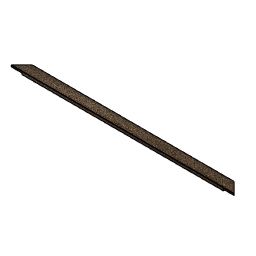
Top_Long (Autodesk Fusion 360 design; units mm, degrees)
Autodesk Fusion 360 part; units mm, degrees
sketch "Sketch1" plane through (0, 0, 0) normal (0, 0, 1) x (1, 0, 0)
  line L0 (914.4, 44.45) -> (914.4, -44.45) construction
  line L1 (914.4, -44.45) -> (-914.4, -44.45)
  line L2 (-914.4, -44.45) -> (-914.4, 44.45) construction
  line L3 (-914.4, 44.45) -> (914.4, -44.45) construction
  line L4 (914.4, 44.45) -> (-914.4, -44.45) construction
  line L5 (-914.4, -44.45) -> (-825.5, 44.45)
  line L6 (914.4, -44.45) -> (825.5, 44.45)
  line L7 (-914.4, 44.45) -> (-825.5, 44.45) construction
  line L8 (825.5, 44.45) -> (914.4, 44.45) construction
  line L9 (-825.5, 44.45) -> (825.5, 44.45)
  line L10 (0, 0) -> (0, -44.45) construction
  dimension "d27" = 1828.8
  dimension "d40" = 45
  dimension "d41" = 45
  dimension "d42" = 88.9
  constraint horizontal L7
  constraint perpendicular L0 L7
  constraint parallel L1 L7
  constraint parallel L0 L2
  constraint coincident L3 L10.start
  constraint coincident L4 L10.start
  constraint coincident L10.start origin
  constraint coincident L6.end L7
  constraint midpoint L1 L10.end
  constraint perpendicular L1 L10
  measures "d27" distance of L0.end L1.end
  measures "d40" angle of L1 L5
  measures "d41" angle of L1 L6
  measures "d42" distance of L1 L9
extrude "Extrude1" add sketch "Sketch1" along normal blind 25.4
sketch "Sketch9" plane through (0, 0, 0) normal (0, 0, 1) x (-1, 0, 0)
  line L0 (825.5, -44.45) -> (914.4, 44.45)
  line L1 (914.4, 44.45) -> (-914.4, 44.45)
  line L2 (-914.4, 44.45) -> (-825.5, -44.45)
  line L3 (914.4, 44.45) -> (825.5, -44.45)
  line L4 (825.5, -44.45) -> (825.5, 44.45)
  line L5 (825.5, 44.45) -> (914.4, 44.45)
  line L6 (-825.5, -44.45) -> (-914.4, 44.45)
  line L7 (-825.5, -44.45) -> (-825.5, 44.45)
  line L8 (-825.5, 44.45) -> (-914.4, 44.45)
  line L9 (-825.5, -44.45) -> (825.5, -44.45)
  line L10 (-825.5, -44.45) -> (-914.4, 44.45)
  line L11 (-914.4, 44.45) -> (914.4, 44.45)
  line L12 (914.4, 44.45) -> (825.5, -44.45)
  line L13 (825.5, -44.45) -> (-825.5, -44.45)
  constraint coincident L0.end L1.start
  constraint coincident L0.start L3.end
  constraint coincident L1 L4.end
  constraint perpendicular L1 L4
  constraint coincident L2.end L6.start
  constraint coincident L1.end L2.start
  constraint coincident L1 L7.end
  constraint perpendicular L1 L7
extrude "Extrude8" cut sketch "Sketch9" along normal blind 12.7 contours L0 L1 L3 L4 L5 L11 L12 | L1 L2 L6 L7 L8 L10 L11
chamfer "Chamfer2" distance 1.5875 angle 45 5 edges at (0, -44.45, 25.4) (0, -44.45, 0) (0, 44.45, 25.4) (914.4, -44.45, 19.05) (-914.4, -44.45, 19.05)
sketch "Sketch11" plane through (0, 44.45, 0) normal (0, 1, 0) x (-1, 0, 0)
  line L0 (825.5, 23.8125) -> (-825.5, 23.8125)
  line L1 (-825.5, 23.8125) -> (-825.5, 12.7)
  line L2 (-825.5, 12.7) -> (-825.5, 0)
  line L3 (-825.5, 0) -> (825.5, 0)
  line L4 (825.5, 0) -> (825.5, 12.7)
  line L5 (825.5, 12.7) -> (825.5, 23.8125)
  line L6 (0, 0) -> (30.1625, 0)
  line L7 (0, 0) -> (-30.1625, 0)
  line L8 (0, 0) -> (0, 12.7) construction
  arc A0 (30.1625, 0) -> (-30.1625, 0) centre (0, -29.468) ccw
  line L9 (-609.6, 0) -> (-609.6, 12.7) construction
  line L10 (-609.6, 0) -> (-579.4375, 0)
  line L11 (-609.6, 0) -> (-639.7625, 0)
  arc A1 (-579.4375, 0) -> (-639.7625, 0) centre (-609.6, -29.468) ccw
  line L12 (-304.8, 0) -> (-304.8, 12.7) construction
  line L13 (-304.8, 0) -> (-274.6375, 0)
  line L14 (-304.8, 0) -> (-334.9625, 0)
  arc A2 (-274.6375, 0) -> (-334.9625, 0) centre (-304.8, -29.468) ccw
  line L15 (304.8, 0) -> (304.8, 12.7) construction
  line L16 (304.8, 0) -> (334.9625, 0)
  line L17 (304.8, 0) -> (274.6375, 0)
  arc A3 (334.9625, 0) -> (274.6375, 0) centre (304.8, -29.468) ccw
  line L18 (609.6, 0) -> (609.6, 12.7) construction
  line L19 (609.6, 0) -> (639.7625, 0)
  line L20 (609.6, 0) -> (579.4375, 0)
  arc A4 (639.7625, 0) -> (579.4375, 0) centre (609.6, -29.468) ccw
  point P0 (-609.6, 0)
  point P1 (-304.8, 0)
  point P2 (304.8, 0)
  point P3 (609.6, 0)
  dimension "d59" = 60.325
  dimension "d60" = 12.7
  dimension "d63" = 304.8
  dimension "d64" = 0
  constraint coincident L6.start L7.start
  constraint coincident L3 L6.end
  constraint parallel L3 L6
  constraint coincident L3 L7.end
  constraint parallel L3 L7
  constraint equal L6 L7
  constraint perpendicular L7 L8
  constraint coincident L8.end A0
  measures "d59" distance of L6.end L7.end
  measures "d60" distance of L6.start L8.end
extrude "Extrude10" cut sketch "Sketch11" against normal blind 3.7703 from surface at -12.7 contours L3 L19 L20 A4 | L3 L10 L11 A1 | L3 L16 L17 A3 | L3 L13 L14 A2 | L3 L6 L7 A0
equation "d59 = 2 in + ( 3 / 8 ) * 1 in"
equation "d66 = ( -19 / 128 ) * 1 in"
